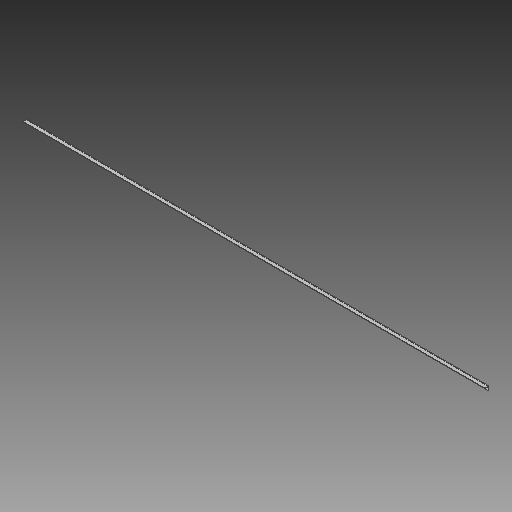
# Autodesk Inventor part: gusset_plate_leftRight
Saved by Autodesk Inventor 2019 (Build 230136000, 136)
## iProperties
Created: 2018-07-11
Part Number: gusset_plate_leftRight
Material: Generic
Document SubType Name: Modeling
Designer: User
Density: 1 g/cm^3
Appearance: Aluminum - Polished
Author: User
Autodesk Inventor part; units mm, degrees
ref_plane "YZ Plane" through (0, 0, 0) normal (1, 0, 0) x (0, 1, 0)
ref_plane "XZ Plane" through (0, 0, 0) normal (0, 1, 0) x (-1, 0, 0)
ref_plane "XY Plane" through (0, 0, 0) normal (0, 0, 1) x (1, 0, 0)
sketch "Sketch1" plane through (0, 0, 0) normal (1, 0, 0) x (0, 1, 0)
  line L0 (0, 0) -> (3.175, 0)
  line L1 (3.175, 0) -> (3.175, -25.4)
  line L2 (3.175, -25.4) -> (-22.225, -25.4)
  line L3 (-22.225, -25.4) -> (-22.225, -22.225)
  line L4 (-22.225, -22.225) -> (0, -22.225)
  line L5 (0, -22.225) -> (0, 0)
  dimension "d0" = 3.175
  dimension "d1" = 3.175
  dimension "d2" = 25.4
  dimension "d3" = 25.4
  constraints: 12 end point, 5 perpendicular, 1 horizontal
  measures "d0" distance of L0.start L0.end
  measures "d1" distance of L2.end L3.end
  measures "d2" distance of L0.end L1.end
  measures "d3" distance of L1.end L2.end
extrude "Extrusion1" add sketch "Sketch1" along normal blind 2997.2
equation "\"wallThick\" = 44.45"
equation "\"roomWidth\" = 3048"
equation "\"roomDepth\" = 3657.6"
equation "\"roomHeight\" = 2438.4"
equation "\"doorWidth\" = 895.35"
equation "\"doorHeight\" = 2108.2"
equation "\"doorX\" = 774.7"
equation "\"doorY\" = 88.9"
equation "\"doorLip\" = 76.2"
equation "\"doorThick\" = 57.15"
equation "\"tubeD\" = 19.05"
equation "\"tubeTurnR\" = 76.2"
body "Solid1"
